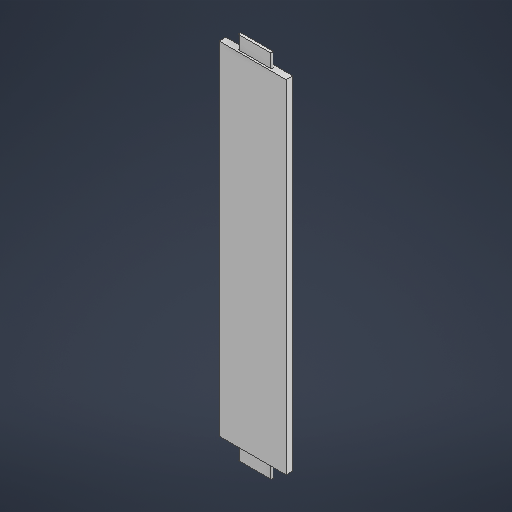
# Autodesk Inventor part: Part3
Saved by Autodesk Inventor 2026.2 (Build 302298010, 298A)
## iProperties
Created: 2026-03-02
Part Number: Part3
Material: Generic
Document SubType Name: Modeling
Designer: shahd
Density: 1 g/cm^3
Appearance: Default
Author: shahd
Autodesk Inventor part; units mm, degrees
ref_plane "YZ Plane" through (0, 0, 0) normal (1, 0, 0) x (0, 1, 0)
ref_plane "XZ Plane" through (0, 0, 0) normal (0, 1, 0) x (-1, 0, 0)
ref_plane "XY Plane" through (0, 0, 0) normal (0, 0, 1) x (1, 0, 0)
sketch "Sketch1" plane through (0, 0, 0) normal (0, 0, 1) x (1, 0, 0)
  line L0 (0, 0) -> (50, 0)
  line L1 (50, 0) -> (50, 255.203)
  line L2 (50, 255.203) -> (0, 255.203)
  line L3 (0, 255.203) -> (0, 0)
  dimension "d0" = 50
  dimension "d1" = 255.203
  constraints: 8 end point, 2 parallel, 1 horizontal, 1 perpendicular
  measures "d0" distance of L2.end L1.end
  measures "d1" distance of L1.end L0.end
extrude "Extrusion1" add sketch "Sketch1" along normal blind 5
sketch "Sketch2" plane through (0, 0, 0) normal (0, -1, 0) x (1, 0, 0)
  line L0 (36.5, 2.5) -> (13.5, 2.5) construction
  line L1 (36.5, 3.5) -> (13.5, 3.5)
  line L2 (13.5, 1.5) -> (36.5, 1.5)
  arc A0 (36.5, 1.5) -> (36.5, 3.5) centre (36.5, 2.5) ccw
  arc A1 (13.5, 3.5) -> (13.5, 1.5) centre (13.5, 2.5) ccw
  line L3 (50, 0) -> (50, 5) projected
  point P0 (0, 0)
  point P1 (25, 2.5)
  point P2 (50, 2.5)
  point P3 (12.5, 2.5)
  point P4 (37.5, 2.5)
  dimension "d4" = 2
  dimension "d5" = 25
  dimension "d6" = 25
  dimension "d9" = 2.5
  constraints: 8 end point, 6 point on circle, 4 tangent, 2 centre point, 2 midpoint, 1 horizontal, 1 parallel
  measures "d4" diameter of A1
  measures "d5" distance of point (50, 2.5) point (25, 2.5)
  measures "d6" distance of point (12.5, 2.5) point (37.5, 2.5)
  measures "d9" vertical distance of point (0, 0) point (25, 2.5)
extrude "Extrusion2" add sketch "Sketch2" along normal blind 10
sketch "Sketch3" plane through (0, 255.203, 0) normal (0, 1, 0) x (1, 0, 0)
  line L0 (36.5, -2.5) -> (13.5, -2.5) construction
  line L1 (36.5, -1.5) -> (13.5, -1.5)
  line L2 (13.5, -3.5) -> (36.5, -3.5)
  arc A0 (36.5, -3.5) -> (36.5, -1.5) centre (36.5, -2.5) ccw
  arc A1 (13.5, -1.5) -> (13.5, -3.5) centre (13.5, -2.5) ccw
  point P0 (0, 0)
  point P1 (25, -2.5)
  point P2 (12.5, -2.5)
  point P3 (37.5, -2.5)
  dimension "d10" = 2
  dimension "d12" = 25
  dimension "d14" = 2.5
  dimension "d15" = 25
  constraints: 8 end point, 6 point on circle, 4 tangent, 2 centre point, 1 horizontal, 1 midpoint, 1 parallel
  measures "d10" diameter of A1
  measures "d12" distance of point (12.5, -2.5) point (37.5, -2.5)
  measures "d14" vertical distance of point (0, 0) point (25, -2.5)
  measures "d15" horizontal distance of point (0, 0) point (25, -2.5)
extrude "Extrusion3" add sketch "Sketch3" along normal blind 10
body "Solid1"
